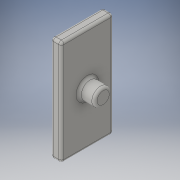
# Autodesk Inventor part: 10x20-sample-bottom-V1
Saved by Autodesk Inventor 2016 (Build 200138000, 138)
## iProperties
Created: 2018-09-09
Part Number: 10x20-sample-bottom-V1
Material: Generic
Document SubType Name: Modeling
Designer: voigt
Density: 1 g/cm^3
Appearance: Default
Author: voigt
Autodesk Inventor part; units mm, degrees
ref_plane "YZ Plane" through (0, 0, 0) normal (1, 0, 0) x (0, 1, 0)
ref_plane "XZ Plane" through (0, 0, 0) normal (0, 1, 0) x (-1, 0, 0)
ref_plane "XY Plane" through (0, 0, 0) normal (0, 0, 1) x (1, 0, 0)
sketch "Sketch1" plane through (0, 0, 0) normal (1, 0, 0) x (0, 1, 0)
  line L0 (0, 13.93) -> (0, -13.93) construction
  line L1 (-6.93, 0) -> (6.93, 0) construction
  line L2 (4.95, 9.95) -> (-4.95, 9.95)
  line L3 (-4.95, 9.95) -> (-4.95, -9.95)
  line L4 (-4.95, -9.95) -> (4.95, -9.95)
  line L5 (4.95, -9.95) -> (4.95, 9.95)
  point P0 (0, 0)
  dimension "d0" = 9.9
  dimension "d1" = 19.9
  constraints: 8 end point, 2 parallel, 1 horizontal, 1 perpendicular, 2 other
  measures "d0" distance of L2.start L2.end
  measures "d1" distance of L4.end L2.start
extrude "Extrusion1" add sketch "Sketch1" along normal blind 2
sketch "Sketch2" plane through (2, 0, 0) normal (1, 0, 0) x (0, 0, -1)
  circle A0 centre (0, 0) radius 1.65
  dimension "d4" = 3.3
  constraints: 1 centre point, 1 coincident
  measures "d4" diameter of A0
extrude "Extrusion2" add sketch "Sketch2" along normal blind 3
fillet "Fillet1" radius 0.5 2 edges at (2, 0, 1.65) (5, 0, 1.65)
fillet "Fillet2" radius 0.5 12 edges at (2, -4.95, 0) (2, 0, 9.95) (1, -4.95, 9.95) (0, -4.95, 0) (1, -4.95, -9.95) (2, 0, -9.95) (0, 0, -9.95) (1, 4.95, -9.95) (0, 4.95, 0) (2, 4.95, 0) (1, 4.95, 9.95) (0, 0, 9.95)
body "Solid1"
